Autodesk Inventor part; units mm, degrees
(part 4 of 5)
  arc A1726 (38.138, -15.9154) -> (38.5736, -15.5159) centre (32.062, -8.8527) ccw
  arc A1727 (38.5736, -15.5159) -> (39.0378, -15.0415) centre (28.2371, -4.9387) ccw
  arc A1728 (39.4893, -14.5664) -> (39.0378, -15.0415) centre (69.1048, -43.1656) ccw
  arc A1729 (39.8856, -14.1661) -> (39.4893, -14.5664) centre (55.6999, -30.2207) ccw
  arc A1730 (40.2317, -13.8281) -> (39.8856, -14.1661) centre (79.9781, -54.8675) ccw
  arc A1731 (40.296, -13.8021) -> (40.2317, -13.8281) centre (40.296, -13.8945) ccw
  arc A1732 (40.3238, -13.8373) -> (40.296, -13.8021) centre (40.296, -13.8306) ccw
  arc A1733 (40.2361, -14.1843) -> (40.3238, -13.8373) centre (23.2158, -9.7) ccw
  arc A1734 (40.1155, -14.6043) -> (40.2361, -14.1843) centre (30.6472, -11.658) ccw
  arc A1735 (39.9532, -15.1035) -> (40.1155, -14.6043) centre (20.5263, -8.5085) ccw
  line L90 (39.9532, -15.1035) -> (39.5114, -16.4048)
  line L91 (39.5114, -16.4048) -> (37.0556, -16.4773)
  arc A1736 (34.2634, -16.5112) -> (37.0556, -16.4773) centre (34.6839, 63.8924) ccw
  arc A1737 (33.9109, -16.1475) -> (34.2634, -16.5112) centre (34.2653, -16.1567) ccw
  arc A1738 (34.1876, -15.4924) -> (33.9109, -16.1475) centre (34.8846, -16.1728) ccw
  arc A1739 (37.1593, -12.4821) -> (34.1876, -15.4924) centre (301.3137, -276.224) ccw
  arc A1740 (37.1593, -12.4821) -> (38.6012, -11.0205) centre (-83.7235, 108.212) ccw
  arc A1741 (38.6012, -11.0205) -> (39.8159, -9.7502) centre (-27.3085, 53.2232) ccw
  arc A1742 (39.8159, -9.7502) -> (40.8574, -8.6344) centre (-176.4109, 193.1049) ccw
  arc A1743 (40.8574, -8.6344) -> (40.9209, -8.4725) centre (40.683, -8.4725) ccw
  arc A1744 (40.9209, -8.4725) -> (40.8525, -8.4427) centre (40.8802, -8.4725) ccw
  arc A1745 (40.8525, -8.4427) -> (39.7666, -9.4542) centre (214.237, -195.6686) ccw
  arc A1746 (39.7666, -9.4542) -> (38.4985, -10.6666) centre (99.0318, -72.7087) ccw
  arc A1747 (38.4985, -10.6666) -> (36.9912, -12.1544) centre (166.2662, -141.6192) ccw
  line L92 (36.9912, -12.1544) -> (33.0615, -16.0783)
  line L93 (33.0615, -16.0783) -> (31.7577, -15.4176)
  line L94 (31.7577, -15.4176) -> (30.454, -14.757)
  line L95 (30.454, -14.757) -> (32.403, -12.6971)
  arc A1748 (33.3514, -11.7342) -> (32.403, -12.6971) centre (56.8365, -35.8159) ccw
  arc A1749 (34.1156, -11.0538) -> (33.3514, -11.7342) centre (41.2243, -19.8071) ccw
  arc A1750 (34.7535, -10.5962) -> (34.1156, -11.0538) centre (38.2519, -16.147) ccw
  arc A1751 (35.297, -10.3468) -> (34.7535, -10.5962) centre (35.964, -12.5169) ccw
  arc A1752 (35.297, -10.3468) -> (35.6895, -10.225) centre (12.0441, 65.3116) ccw
  arc A1753 (35.6895, -10.225) -> (36.0874, -10.0994) centre (10.5624, 70.0447) ccw
  arc A1754 (36.0874, -10.0994) -> (36.4381, -9.9868) centre (13.3316, 61.3495) ccw
  arc A1755 (36.4381, -9.9868) -> (36.6604, -9.9126) centre (32.3763, 2.5531) ccw
  arc A1756 (36.7054, -9.9776) -> (36.6604, -9.9126) centre (36.6738, -9.9514) ccw
  arc A1757 (36.1561, -10.6219) -> (36.7054, -9.9776) centre (16.3124, 6.8533) ccw
  arc A1758 (35.3718, -11.4796) -> (36.1561, -10.6219) centre (12.8473, 9.9048) ccw
  arc A1759 (34.3562, -12.5291) -> (35.3718, -11.4796) centre (-20.1635, 41.2446) ccw
  arc A1760 (34.3562, -12.5291) -> (33.3301, -13.588) centre (93.5068, -70.8702) ccw
  arc A1761 (33.3301, -13.588) -> (32.509, -14.4785) centre (60.9355, -39.8655) ccw
  arc A1762 (32.509, -14.4785) -> (31.8583, -15.2176) centre (84.1452, -60.5934) ccw
  arc A1763 (31.8583, -15.2176) -> (31.8911, -15.2894) centre (31.8911, -15.246) ccw
  arc A1764 (31.8911, -15.2894) -> (32.059, -15.2242) centre (31.8911, -15.0404) ccw
  arc A1765 (32.059, -15.2242) -> (32.9062, -14.4424) centre (-48.4152, 72.8292) ccw
  arc A1766 (32.9062, -14.4424) -> (33.8794, -13.5112) centre (-1.8359, 22.8417) ccw
  arc A1767 (33.8794, -13.5112) -> (34.9854, -12.406) centre (-30.7449, 52.2666) ccw
  arc A1768 (36.9022, -10.5345) -> (34.9854, -12.406) centre (82.5718, -59.2267) ccw
  arc A1769 (38.4555, -9.2015) -> (36.9022, -10.5345) centre (52.7577, -27.4394) ccw
  arc A1770 (39.6868, -8.3356) -> (38.4555, -9.2015) centre (47.371, -20.5704) ccw
  arc A1771 (40.4694, -8.1054) -> (39.6868, -8.3356) centre (40.4864, -9.6088) ccw
  arc A1772 (40.657, -8.1316) -> (40.4694, -8.1054) centre (40.4766, -8.7387) ccw
  arc A1773 (40.8777, -8.2165) -> (40.657, -8.1316) centre (40.227, -9.5787) ccw
  arc A1774 (41.0953, -8.3415) -> (40.8777, -8.2165) centre (40.1633, -9.7121) ccw
  arc A1775 (41.275, -8.4902) -> (41.0953, -8.3415) centre (40.3973, -9.3679) ccw
  arc A1776 (31.7084, -10.6223) -> (31.7492, -10.5098) centre (31.5736, -10.5098) ccw
  arc A1777 (31.3694, -11.0202) -> (31.7084, -10.6223) centre (11.4621, 6.2854) ccw
  arc A1778 (30.9517, -11.4825) -> (31.3694, -11.0202) centre (19.0472, -0.3084) ccw
  arc A1779 (30.4563, -11.9971) -> (30.9517, -11.4825) centre (10.4353, 7.7752) ccw
  arc A1780 (30.4563, -11.9971) -> (29.9776, -12.4996) centre (44.1557, -25.5264) ccw
  arc A1781 (29.9776, -12.4996) -> (29.6159, -12.9217) centre (35.8733, -17.9166) ccw
  arc A1782 (29.6159, -12.9217) -> (29.3775, -13.2419) centre (34.2682, -16.6353) ccw
  arc A1783 (29.3775, -13.2419) -> (29.4112, -13.3063) centre (29.4112, -13.2653) ccw
  arc A1784 (29.4112, -13.3063) -> (29.5618, -13.2534) centre (29.4112, -13.0654) ccw
  arc A1785 (29.5618, -13.2534) -> (29.9818, -12.9058) centre (18.97, -0.0287) ccw
  arc A1786 (29.9818, -12.9058) -> (30.4717, -12.4653) centre (21.3967, -2.8664) ccw
  arc A1787 (30.4717, -12.4653) -> (31.0055, -11.9429) centre (15.5086, 3.3615) ccw
  arc A1788 (31.7567, -11.2175) -> (31.0055, -11.9429) centre (46.6591, -27.402) ccw
  arc A1789 (32.2629, -10.8345) -> (31.7567, -11.2175) centre (33.9908, -13.6438) ccw
  arc A1790 (32.7105, -10.6444) -> (32.2629, -10.8345) centre (33.1169, -12.223) ccw
  arc A1791 (33.2222, -10.5796) -> (32.7105, -10.6444) centre (33.2222, -12.6321) ccw
  line L96 (33.2222, -10.5796) -> (34.0925, -10.5796)
  line L97 (34.0925, -10.5796) -> (32.1196, -12.5641)
  arc A1792 (31.3452, -13.3188) -> (32.1196, -12.5641) centre (7.8652, 11.548) ccw
  arc A1793 (30.6521, -13.9417) -> (31.3452, -13.3188) centre (18.3556, 0.438) ccw
  arc A1794 (30.058, -14.4365) -> (30.6521, -13.9417) centre (11.4069, 8.5638) ccw
  arc A1795 (29.8944, -14.4669) -> (30.058, -14.4365) centre (29.9482, -14.301) ccw
  arc A1796 (29.7762, -14.393) -> (29.8944, -14.4669) centre (29.9829, -14.1937) ccw
  arc A1797 (29.6203, -14.2122) -> (29.7762, -14.393) centre (31.3225, -12.9019) ccw
  arc A1798 (29.459, -13.9774) -> (29.6203, -14.2122) centre (31.6971, -12.6135) ccw
  arc A1799 (29.3154, -13.7147) -> (29.459, -13.9774) centre (32.1853, -12.316) ccw
  arc A1800 (29.1585, -13.0704) -> (29.3154, -13.7147) centre (30.7144, -13.0329) ccw
  arc A1801 (29.236, -12.262) -> (29.1585, -13.0704) centre (32.5603, -12.9883) ccw
  arc A1802 (29.5153, -11.4435) -> (29.236, -12.262) centre (32.9572, -13.075) ccw
  arc A1803 (29.9598, -10.7655) -> (29.5153, -11.4435) centre (32.1847, -12.7089) ccw
  arc A1804 (30.3493, -10.5014) -> (29.9598, -10.7655) centre (30.657, -11.3745) ccw
  arc A1805 (30.9913, -10.344) -> (30.3493, -10.5014) centre (31.4668, -13.6724) ccw
  arc A1806 (31.5755, -10.3233) -> (30.9913, -10.344) centre (31.3801, -13.0655) ccw
  arc A1807 (31.7492, -10.5098) -> (31.5755, -10.3233) centre (31.5622, -10.5098) ccw
  arc A1808 (46.7213, -8.0425) -> (46.3577, -8.3987) centre (47.4846, -9.1857) ccw
  arc A1809 (46.3577, -8.3987) -> (46.1142, -8.8903) centre (47.8654, -9.4516) ccw
  arc A1810 (46.1142, -8.8903) -> (46.0266, -9.4315) centre (47.8632, -9.4509) ccw
  arc A1811 (46.0266, -9.4315) -> (46.1158, -9.9317) centre (47.3936, -9.4459) ccw
  arc A1812 (46.1158, -9.9317) -> (46.4364, -10.4266) centre (47.4287, -9.4326) ccw
  arc A1813 (46.4364, -10.4266) -> (46.9984, -10.8648) centre (48.4994, -8.36) ccw
  arc A1814 (46.9984, -10.8648) -> (47.6192, -11.1375) centre (48.3863, -8.5487) ccw
  arc A1815 (47.6192, -11.1375) -> (48.1096, -11.1265) centre (47.8471, -10.3684) ccw
  arc A1816 (48.1096, -11.1265) -> (48.8176, -10.6423) centre (47.5768, -9.5875) ccw
  arc A1817 (48.8176, -10.6423) -> (49.2477, -9.8286) centre (47.1986, -9.266) ccw
  arc A1818 (49.2477, -9.8286) -> (49.2809, -8.9454) centre (47.3812, -9.3162) ccw
  arc A1819 (49.2809, -8.9454) -> (48.8957, -8.2631) centre (48.0631, -9.1831) ccw
  arc A1820 (48.8957, -8.2631) -> (48.4527, -8.0069) centre (48.077, -9.1676) ccw
  arc A1821 (48.4527, -8.0069) -> (47.8163, -7.8732) centre (47.5061, -10.9318) ccw
  arc A1822 (47.8163, -7.8732) -> (47.1752, -7.8767) centre (47.5119, -10.8742) ccw
  arc A1823 (47.1752, -7.8767) -> (46.7213, -8.0425) centre (47.2894, -8.8933) ccw
  arc A1824 (48.7931, -8.8222) -> (48.5558, -8.3982) centre (47.9232, -9.0307) ccw
  arc A1825 (48.8362, -9.4068) -> (48.7931, -8.8222) centre (47.0228, -9.2466) ccw
  arc A1826 (48.6892, -9.9974) -> (48.8362, -9.4068) centre (46.8825, -9.2342) ccw
  arc A1827 (48.3754, -10.4393) -> (48.6892, -9.9974) centre (47.5338, -9.5093) ccw
  arc A1828 (48.087, -10.6623) -> (48.3754, -10.4393) centre (46.7951, -8.6931) ccw
  arc A1829 (47.8597, -10.7406) -> (48.087, -10.6623) centre (47.8192, -10.254) ccw
  arc A1830 (47.6028, -10.7066) -> (47.8597, -10.7406) centre (47.8092, -10.1344) ccw
  arc A1831 (47.198, -10.5374) -> (47.6028, -10.7066) centre (49.0977, -6.5617) ccw
  arc A1832 (46.9119, -10.3629) -> (47.198, -10.5374) centre (47.9066, -9.0545) ccw
  arc A1833 (46.6708, -10.1357) -> (46.9119, -10.3629) centre (47.8627, -9.1122) ccw
  arc A1834 (46.4984, -9.8815) -> (46.6708, -10.1357) centre (47.6992, -9.2526) ccw
  arc A1835 (46.4164, -9.6272) -> (46.4984, -9.8815) centre (47.1954, -9.5165) ccw
  arc A1836 (46.5581, -8.8824) -> (46.4164, -9.6272) centre (47.5771, -9.4622) ccw
  arc A1837 (47.1366, -8.3016) -> (46.5581, -8.8824) centre (47.9132, -9.6534) ccw
  arc A1838 (47.9043, -8.113) -> (47.1366, -8.3016) centre (47.8475, -9.5391) ccw
  arc A1839 (48.5558, -8.3982) -> (47.9043, -8.113) centre (47.8655, -9.0885) ccw
  arc A1840 (-50.4415, -11.5045) -> (-50.7344, -11.3634) centre (-51.3001, -12.9124) ccw
  arc A1841 (-50.2214, -11.6868) -> (-50.4415, -11.5045) centre (-50.9596, -12.354) ccw
  arc A1842 (-50.0815, -11.9045) -> (-50.2214, -11.6868) centre (-50.8108, -12.2195) ccw
  arc A1843 (-50.024, -12.1495) -> (-50.0815, -11.9045) centre (-50.737, -12.1877) ccw
  arc A1844 (-50.024, -12.1495) -> (-50.0042, -12.4881) centre (-14.2029, -10.2317) ccw
  arc A1845 (-50.0042, -12.4881) -> (-49.98, -12.5211) centre (-49.9665, -12.4857) ccw
  arc A1846 (-49.98, -12.5211) -> (-49.9513, -12.5064) centre (-49.9722, -12.5008) ccw
  arc A1847 (-49.9513, -12.5064) -> (-49.8731, -12.2072) centre (-74.3795, -5.9632) ccw
  arc A1848 (-49.8731, -12.2072) -> (-49.9017, -11.8206) centre (-50.4639, -12.0567) ccw
  arc A1849 (-49.9017, -11.8206) -> (-50.1607, -11.4431) centre (-50.9451, -12.2587) ccw
  arc A1850 (-50.1607, -11.4431) -> (-50.5726, -11.1738) centre (-51.0791, -12.3981) ccw
  arc A1851 (-50.5726, -11.1738) -> (-51.0297, -11.0949) centre (-50.9763, -12.1494) ccw
  arc A1852 (-51.0297, -11.0949) -> (-51.1035, -11.1276) centre (-51.024, -11.2076) ccw
  arc A1853 (-51.1035, -11.1276) -> (-51.1023, -11.1819) centre (-51.0771, -11.1541) ccw
  arc A1854 (-51.1023, -11.1819) -> (-50.9743, -11.2658) centre (-50.7742, -10.8211) ccw
  arc A1855 (-50.9743, -11.2658) -> (-50.7344, -11.3634) centre (-49.511, -8.0137) ccw
  arc A1856 (-8.6486, -11.8882) -> (-9.2341, -12.3218) centre (-7.6704, -13.8214) ccw
  arc A1857 (-9.2341, -12.3218) -> (-9.814, -13.0398) centre (-5.3124, -16.0826) ccw
  arc A1858 (-9.814, -13.0398) -> (-10.2534, -13.8266) centre (-5.4203, -16.0096) ccw
  arc A1859 (-10.2534, -13.8266) -> (-10.3912, -14.4664) centre (-8.8369, -14.4664) ccw
  arc A1860 (-10.3912, -14.4664) -> (-10.2891, -15.198) centre (-7.718, -14.4664) ccw
  arc A1861 (-10.2891, -15.198) -> (-9.9826, -15.9905) centre (-5.8322, -13.9298) ccw
  arc A1862 (-9.9826, -15.9905) -> (-9.5475, -16.6938) centre (-6.0016, -14.0139) ccw
  arc A1863 (-9.5475, -16.6938) -> (-9.058, -17.1515) centre (-7.9836, -15.5118) ccw
  arc A1864 (-9.058, -17.1515) -> (-8.277, -17.522) centre (-7.3254, -14.5073) ccw
  arc A1865 (-8.277, -17.522) -> (-7.3739, -17.6972) centre (-7.0611, -13.67) ccw
  arc A1866 (-7.3739, -17.6972) -> (-6.476, -17.6621) centre (-7.0747, -13.8454) ccw
  arc A1867 (-6.476, -17.6621) -> (-5.7108, -17.4116) centre (-6.8656, -15.1784) ccw
  arc A1868 (-5.7108, -17.4116) -> (-4.7772, -16.6666) centre (-7.1175, -14.6913) ccw
  arc A1869 (-4.7772, -16.6666) -> (-4.1582, -15.5951) centre (-7.4602, -14.4021) ccw
  arc A1870 (-4.1582, -15.5951) -> (-3.9541, -14.3873) centre (-7.3882, -14.4281) ccw
  arc A1871 (-3.9541, -14.3873) -> (-4.2077, -13.2514) centre (-6.7741, -14.4208) ccw
  arc A1872 (-4.2077, -13.2514) -> (-4.9315, -12.3561) centre (-6.3063, -14.2076) ccw
  arc A1873 (-4.9315, -12.3561) -> (-6.1103, -11.7598) centre (-7.2532, -15.4829) ccw
  arc A1874 (-6.1103, -11.7598) -> (-7.4534, -11.5815) centre (-7.3143, -15.6818) ccw
  arc A1875 (-7.4534, -11.5815) -> (-8.6486, -11.8882) centre (-7.3564, -14.4419) ccw
  arc A1876 (-4.7478, -13.2418) -> (-5.2538, -12.6927) centre (-11.7267, -19.1656) ccw
  arc A1877 (-4.5289, -13.6208) -> (-4.7478, -13.2418) centre (-5.6794, -14.0326) ccw
  arc A1878 (-4.4572, -14.0533) -> (-4.5289, -13.6208) centre (-5.6855, -14.0347) ccw
  arc A1879 (-4.4988, -14.8023) -> (-4.4572, -14.0533) centre (-13.7563, -13.9127) ccw
  arc A1880 (-4.6776, -15.7395) -> (-4.4988, -14.8023) centre (-9.6283, -14.3094) ccw
  arc A1881 (-5.0155, -16.4236) -> (-4.6776, -15.7395) centre (-6.7527, -15.1401) ccw
  arc A1882 (-5.5524, -16.9186) -> (-5.0155, -16.4236) centre (-6.5733, -15.2726) ccw
  arc A1883 (-6.3311, -17.2823) -> (-5.5524, -16.9186) centre (-7.4731, -13.8219) ccw
  arc A1884 (-7.6809, -17.3654) -> (-6.3311, -17.2823) centre (-7.1637, -14.7594) ccw
  arc A1885 (-8.8938, -16.7727) -> (-7.6809, -17.3654) centre (-7.1671, -14.7764) ccw
  arc A1886 (-9.6718, -15.6457) -> (-8.8938, -16.7727) centre (-7.1073, -14.7072) ccw
  arc A1887 (-9.8229, -14.2621) -> (-9.6718, -15.6457) centre (-6.9455, -14.648) ccw
  arc A1888 (-9.5204, -13.2273) -> (-9.8229, -14.2621) centre (-6.2735, -14.7382) ccw
  arc A1889 (-8.9428, -12.4702) -> (-9.5204, -13.2273) centre (-7.5078, -14.1638) ccw
  arc A1890 (-8.0839, -12.0074) -> (-8.9428, -12.4702) centre (-7.4209, -14.2664) ccw
  arc A1891 (-6.958, -11.8347) -> (-8.0839, -12.0074) centre (-6.8769, -16.1196) ccw
  arc A1892 (-6.5115, -11.8746) -> (-6.958, -11.8347) centre (-6.9186, -13.9142) ccw
  arc A1893 (-6.1183, -12.01) -> (-6.5115, -11.8746) centre (-6.8146, -13.393) ccw
  arc A1894 (-5.7208, -12.269) -> (-6.1183, -12.01) centre (-7.0812, -13.9226) ccw
  arc A1895 (-5.2538, -12.6927) -> (-5.7208, -12.269) centre (-9.8548, -17.2937) ccw
  arc A1896 (21.7067, -11.8336) -> (21.1335, -12.2767) centre (22.6164, -13.6027) ccw
  arc A1897 (21.1335, -12.2767) -> (20.6054, -13) centre (24.5132, -15.2988) ccw
  arc A1898 (20.6054, -13) -> (20.2257, -13.8207) centre (24.5692, -15.3317) ccw
  arc A1899 (20.2257, -13.8207) -> (20.1023, -14.561) centre (22.3265, -14.5515) ccw
  arc A1900 (20.1023, -14.561) -> (20.547, -16.1601) centre (23.248, -14.5476) ccw
  arc A1901 (20.547, -16.1601) -> (21.7473, -17.332) centre (23.357, -14.4825) ccw
  arc A1902 (21.7473, -17.332) -> (23.3658, -17.7519) centre (23.3447, -14.5043) ccw
  arc A1903 (23.3658, -17.7519) -> (24.9522, -17.3008) centre (23.3457, -14.6664) ccw
  arc A1904 (24.9522, -17.3008) -> (25.9352, -16.3533) centre (23.3193, -14.623) ccw
  arc A1905 (25.9352, -16.3533) -> (26.4072, -15.0895) centre (23.4348, -14.6994) ccw
  arc A1906 (26.4072, -15.0895) -> (26.2808, -13.7295) centre (23.3481, -14.688) ccw
  arc A1907 (26.2808, -13.7295) -> (25.5804, -12.5135) centre (23.0306, -14.7918) ccw
  arc A1908 (25.5804, -12.5135) -> (25.1593, -12.105) centre (22.5116, -15.2555) ccw
  arc A1909 (25.1593, -12.105) -> (24.7721, -11.8685) centre (24.1861, -13.263) ccw
  arc A1910 (24.7721, -11.8685) -> (24.2922, -11.7358) centre (24.0164, -13.667) ccw
  arc A1911 (24.2922, -11.7358) -> (23.5487, -11.6599) centre (22.9749, -20.9586) ccw
  arc A1912 (23.5487, -11.6599) -> (22.9979, -11.647) centre (23.1056, -18.8402) ccw
  arc A1913 (22.9979, -11.647) -> (22.4536, -11.6767) centre (23.1011, -18.543) ccw
  arc A1914 (22.4536, -11.6767) -> (21.9858, -11.7397) centre (23.0095, -17.571) ccw
  arc A1915 (21.9858, -11.7397) -> (21.7067, -11.8336) centre (22.1555, -12.7063) ccw
  arc A1916 (24.9716, -12.4173) -> (24.4203, -12.0607) centre (23.8629, -13.527) ccw
  arc A1917 (25.5115, -13.0765) -> (24.9716, -12.4173) centre (21.9442, -15.4472) ccw
  arc A1918 (25.9145, -13.8372) -> (25.5115, -13.0765) centre (21.8957, -15.4795) ccw
  arc A1919 (26.0469, -14.5082) -> (25.9145, -13.8372) centre (24.2654, -14.5111) ccw
  arc A1920 (25.9247, -15.2823) -> (26.0469, -14.5082) centre (23.5599, -14.5122) ccw
  arc A1921 (25.5627, -16.0554) -> (25.9247, -15.2823) centre (22.62, -14.2061) ccw
  arc A1922 (25.0239, -16.7157) -> (25.5627, -16.0554) centre (22.6297, -14.2122) ccw
  arc A1923 (24.3818, -17.1579) -> (25.0239, -16.7157) centre (23.3328, -14.9474) ccw
  arc A1924 (23.0524, -17.4187) -> (24.3818, -17.1579) centre (23.2049, -14.6779) ccw
  arc A1925 (21.801, -16.9988) -> (23.0524, -17.4187) centre (23.1908, -14.9316) ccw
  arc A1926 (20.9144, -15.9847) -> (21.801, -16.9988) centre (23.2601, -14.8286) ccw
  arc A1927 (20.5944, -14.6114) -> (20.9144, -15.9847) centre (23.7007, -14.6114) ccw
  arc A1928 (20.6315, -13.9946) -> (20.5944, -14.6114) centre (25.7415, -14.6114) ccw
  arc A1929 (20.7507, -13.5536) -> (20.6315, -13.9946) centre (22.2124, -14.1855) ccw
  arc A1930 (20.9941, -13.1527) -> (20.7507, -13.5536) centre (22.3204, -14.2321) ccw
  arc A1931 (21.4372, -12.6618) -> (20.9941, -13.1527) centre (26.0121, -17.2367) ccw
  arc A1932 (22.1134, -12.1257) -> (21.4372, -12.6618) centre (24.0937, -15.3183) ccw
  arc A1933 (22.8041, -11.8522) -> (22.1134, -12.1257) centre (23.2181, -13.9066) ccw
  arc A1934 (23.5572, -11.834) -> (22.8041, -11.8522) centre (23.2324, -13.9776) ccw
  arc A1935 (24.4203, -12.0607) -> (23.5572, -11.834) centre (22.9282, -15.9853) ccw
  arc A1936 (-61.0775, -12.1557) -> (-61.2696, -12.3511) centre (-60.5776, -12.8394) ccw
  arc A1937 (-61.2696, -12.3511) -> (-61.4156, -12.6202) centre (-60.2017, -13.1046) ccw
  arc A1938 (-61.4156, -12.6202) -> (-61.5073, -12.9461) centre (-59.9224, -13.2161) ccw
  arc A1939 (-61.5073, -12.9461) -> (-61.538, -13.3098) centre (-59.3719, -13.3098) ccw
  arc A1940 (-61.538, -13.3098) -> (-61.2621, -14.2496) centre (-59.7999, -13.3098) ccw
  arc A1941 (-61.2621, -14.2496) -> (-60.5238, -14.8803) centre (-59.8459, -13.3394) ccw
  arc A1942 (-60.5238, -14.8803) -> (-59.5734, -14.9904) centre (-59.8701, -13.3944) ccw
  arc A1943 (-59.5734, -14.9904) -> (-58.7287, -14.5457) centre (-59.8678, -13.4066) ccw
  arc A1944 (-58.7287, -14.5457) -> (-58.283, -13.4563) centre (-59.8049, -13.4695) ccw
  arc A1945 (-58.283, -13.4563) -> (-58.7393, -12.3545) centre (-59.8745, -13.4701) ccw
  arc A1946 (-58.7393, -12.3545) -> (-59.875, -11.8196) centre (-60.0311, -13.624) ccw
  arc A1947 (-59.875, -11.8196) -> (-61.0775, -12.1557) centre (-60.0282, -13.5907) ccw
  arc A1948 (-58.6887, -13.1367) -> (-58.8881, -12.5872) centre (-59.8097, -13.2327) ccw
  arc A1949 (-58.755, -13.7936) -> (-58.6887, -13.1367) centre (-60.4668, -13.2889) ccw
  arc A1950 (-59.0517, -14.3667) -> (-58.755, -13.7936) centre (-60.3851, -13.313) ccw
  arc A1951 (-59.5052, -14.6801) -> (-59.0517, -14.3667) centre (-59.7898, -13.7835) ccw
  arc A1952 (-60.0271, -14.6894) -> (-59.5052, -14.6801) centre (-59.7818, -13.8087) ccw
  arc A1953 (-60.6031, -14.4198) -> (-60.0271, -14.6894) centre (-59.5107, -12.8359) ccw
  arc A1954 (-61.0522, -13.9824) -> (-60.6031, -14.4198) centre (-59.5411, -12.8801) ccw
  arc A1955 (-61.2075, -13.506) -> (-61.0522, -13.9824) centre (-60.3992, -13.506) ccw
  arc A1956 (-60.9619, -12.7146) -> (-61.2075, -13.506) centre (-59.8099, -13.506) ccw
  arc A1957 (-60.3098, -12.1948) -> (-60.9619, -12.7146) centre (-59.7831, -13.5244) ccw
  arc A1958 (-59.5167, -12.1481) -> (-60.3098, -12.1948) centre (-59.8425, -13.3744) ccw
  arc A1959 (-58.8881, -12.5872) -> (-59.5167, -12.1481) centre (-59.8037, -13.2285) ccw
  arc A1960 (-52.0358, -12.548) -> (-52.0178, -12.6484) centre (-51.7463, -12.548) ccw
  arc A1961 (-52.0178, -12.6484) -> (-51.9638, -12.7572) centre (-51.4817, -12.4501) ccw
  arc A1962 (-51.9638, -12.7572) -> (-51.8845, -12.8575) centre (-51.4358, -12.4209) ccw
  arc A1963 (-51.8845, -12.8575) -> (-51.7908, -12.9327) centre (-51.5327, -12.5152) ccw
  arc A1964 (-51.7908, -12.9327) -> (-51.7071, -12.961) centre (-51.688, -12.7665) ccw
  arc A1965 (-51.7071, -12.961) -> (-51.6576, -12.9314) centre (-51.7024, -12.9127) ccw
  arc A1966 (-51.6576, -12.9314) -> (-51.6499, -12.8432) centre (-51.7923, -12.8751) ccw
  arc A1967 (-51.6499, -12.8432) -> (-51.6933, -12.6995) centre (-52.6572, -13.0693) ccw
  arc A1968 (-51.6933, -12.6995) -> (-51.814, -12.4337) centre (-53.9686, -13.5725) ccw
  arc A1969 (-51.814, -12.4337) -> (-51.9264, -12.329) centre (-52.0211, -12.5432) ccw
  arc A1970 (-51.9264, -12.329) -> (-52.0066, -12.3648) centre (-51.9503, -12.3832) ccw
  arc A1971 (-52.0066, -12.3648) -> (-52.0358, -12.548) centre (-51.4456, -12.548) ccw
  arc A1972 (-51.0907, -13.2277) -> (-50.9552, -13.2664) centre (-50.8353, -12.5895) ccw
  arc A1973 (-50.9552, -13.2664) -> (-50.817, -13.2757) centre (-50.8434, -12.6348) ccw
  arc A1974 (-50.817, -13.2757) -> (-50.6967, -13.2561) centre (-50.8378, -12.7693) ccw
  arc A1975 (-50.6967, -13.2561) -> (-50.6156, -13.2082) centre (-50.7493, -13.0745) ccw
  arc A1976 (-50.6156, -13.2082) -> (-50.6042, -13.1539) centre (-50.6515, -13.1722) ccw
  arc A1977 (-50.6042, -13.1539) -> (-50.6494, -13.1081) centre (-50.6794, -13.183) ccw
  arc A1978 (-50.6494, -13.1081) -> (-50.7684, -13.0807) centre (-50.7973, -13.4778) ccw
  arc A1979 (-50.7684, -13.0807) -> (-50.941, -13.078) centre (-50.8786, -14.5925) ccw
  arc A1980 (-50.941, -13.078) -> (-51.126, -13.0926) centre (-50.8399, -15.5323) ccw
  arc A1981 (-51.126, -13.0926) -> (-51.1983, -13.1276) centre (-51.1117, -13.2142) ccw
  arc A1982 (-51.1983, -13.1276) -> (-51.194, -13.1728) centre (-51.1775, -13.1485) ccw
  arc A1983 (-51.194, -13.1728) -> (-51.0907, -13.2277) centre (-50.8892, -12.7241) ccw
  arc A1984 (54.3957, -29.633) -> (53.8937, -29.9822) centre (57.8749, -35.1695) ccw
  arc A1985 (53.8937, -29.9822) -> (53.5183, -30.3224) centre (55.7859, -32.4477) ccw
  arc A1986 (53.5183, -30.3224) -> (53.3673, -30.5575) centre (54.0814, -30.8502) ccw
  arc A1987 (53.3673, -30.5575) -> (53.4348, -30.6582) centre (53.4348, -30.5852) ccw
  arc A1988 (53.4348, -30.6582) -> (53.52, -30.6333) centre (53.4348, -30.5004) ccw
  arc A1989 (53.52, -30.6333) -> (53.6954, -30.5135) centre (51.5661, -27.5843) ccw
  arc A1990 (53.6954, -30.5135) -> (53.8992, -30.3542) centre (51.504, -27.4989) ccw
  arc A1991 (53.8992, -30.3542) -> (54.1126, -30.1655) centre (50.3806, -26.1597) ccw
  arc A1992 (55.6105, -29.4753) -> (54.1126, -30.1655) centre (55.909, -32.0938) ccw
  arc A1993 (57.241, -29.8019) -> (55.6105, -29.4753) centre (55.9181, -32.1732) ccw
  arc A1994 (58.4128, -31.0329) -> (57.241, -29.8019) centre (55.8452, -32.3038) ccw
  arc A1995 (58.6904, -32.7194) -> (58.4128, -31.0329) centre (55.7911, -32.3306) ccw
  arc A1996 (58.4067, -33.7014) -> (58.6904, -32.7194) centre (55.2548, -32.2586) ccw
  arc A1997 (57.8674, -34.4181) -> (58.4067, -33.7014) centre (56.5025, -32.8298) ccw
  arc A1998 (57.0722, -34.849) -> (57.8674, -34.4181) centre (56.4745, -32.7972) ccw
  arc A1999 (56.041, -34.9962) -> (57.0722, -34.849) centre (56.041, -31.3092) ccw
  arc A2000 (55.3527, -34.964) -> (56.041, -34.9962) centre (56.041, -27.61) ccw
  arc A2001 (54.8936, -34.8559) -> (55.3527, -34.964) centre (55.5124, -33.2584) ccw
  arc A2002 (54.4997, -34.6315) -> (54.8936, -34.8559) centre (55.448, -33.4246) ccw
  arc A2003 (54.035, -34.2192) -> (54.4997, -34.6315) centre (57.7167, -30.5374) ccw
  arc A2004 (53.617, -33.7476) -> (54.035, -34.2192) centre (57.744, -30.5101) ccw
  arc A2005 (53.3941, -33.3508) -> (53.617, -33.7476) centre (54.7882, -32.8288) ccw
  arc A2006 (53.2884, -32.8797) -> (53.3941, -33.3508) centre (55.0414, -32.734) ccw
  arc A2007 (53.2579, -32.1438) -> (53.2884, -32.8797) centre (62.1467, -32.1438) ccw
  arc A2008 (53.2579, -32.1438) -> (53.2459, -31.6008) centre (40.9961, -32.1438) ccw
  arc A2009 (53.2459, -31.6008) -> (53.2019, -31.2714) centre (51.3667, -31.6841) ccw
  arc A2010 (53.2019, -31.2714) -> (53.1293, -31.1668) centre (53.0367, -31.3086) ccw
  arc A2011 (53.1293, -31.1668) -> (53.0425, -31.1856) centre (53.0952, -31.219) ccw
  arc A2012 (53.0425, -31.1856) -> (52.8122, -32.0857) centre (54.3121, -31.9899) ccw
  arc A2013 (52.8122, -32.0857) -> (53.0721, -33.2523) centre (56.6656, -31.8396) ccw
  arc A2014 (53.0721, -33.2523) -> (53.7034, -34.3497) centre (57.0808, -31.6763) ccw
  arc A2015 (53.7034, -34.3497) -> (54.562, -35.0509) centre (55.7275, -32.7475) ccw
  arc A2016 (54.562, -35.0509) -> (55.7936, -35.3677) centre (55.8976, -32.4114) ccw
  arc A2017 (55.7936, -35.3677) -> (57.0675, -35.1472) centre (55.9044, -32.2185) ccw
  arc A2018 (57.0675, -35.1472) -> (58.1619, -34.4282) centre (55.8703, -32.1325) ccw
  arc A2019 (58.1619, -34.4282) -> (58.8838, -33.3345) centre (55.864, -32.1263) ccw
  arc A2020 (58.8838, -33.3345) -> (59.1079, -32.7077) centre (50.5845, -30.0138) ccw
  arc A2021 (59.1079, -32.7077) -> (59.1718, -32.3059) centre (57.797, -32.2934) ccw
  arc A2022 (59.1718, -32.3059) -> (59.1146, -31.907) centre (57.836, -32.2937) ccw
  arc A2023 (59.1146, -31.907) -> (58.9024, -31.2943) centre (51.2905, -34.2732) ccw
  arc A2024 (58.9024, -31.2943) -> (58.7043, -30.8741) centre (55.7009, -32.5472) ccw
  arc A2025 (58.7043, -30.8741) -> (58.4351, -30.4451) centre (54.4672, -33.2344) ccw
  arc A2026 (58.4351, -30.4451) -> (58.1399, -30.0696) centre (54.7798, -33.0147) ccw
  arc A2027 (58.1399, -30.0696) -> (57.8652, -29.8188) centre (56.8787, -31.175) ccw
  arc A2028 (57.8652, -29.8188) -> (57.0705, -29.4158) centre (56.2154, -32.0869) ccw
  arc A2029 (57.0705, -29.4158) -> (56.1262, -29.2423) centre (55.9253, -32.993) ccw
  arc A2030 (56.1262, -29.2423) -> (55.184, -29.3146) centre (55.9314, -32.8794) ccw
  arc A2031 (55.184, -29.3146) -> (54.3957, -29.633) centre (55.6789, -31.6749) ccw
  arc A2032 (54.8437, -31.1688) -> (54.6468, -31.385) centre (56.0572, -32.4713) ccw
  arc A2033 (54.6468, -31.385) -> (54.508, -31.6124) centre (55.623, -32.1368) ccw
  arc A2034 (54.508, -31.6124) -> (54.4429, -31.817) centre (55.25, -31.9614) ccw
  arc A2035 (54.4429, -31.817) -> (54.4705, -31.9622) centre (54.6464, -31.8534) ccw
  arc A2036 (54.4705, -31.9622) -> (54.5564, -32.072) centre (55.0097, -31.6289) ccw
  arc A2037 (54.5564, -32.072) -> (54.6292, -32.0918) centre (54.6096, -32.0199) ccw
  arc A2038 (54.6292, -32.0918) -> (54.694, -32.0375) centre (54.6026, -31.994) ccw
  arc A2039 (54.694, -32.0375) -> (54.7524, -31.8854) centre (53.7388, -31.5836) ccw
  arc A2040 (54.8213, -31.7254) -> (54.7524, -31.8854) centre (55.468, -32.0985) ccw
  arc A2041 (54.9428, -31.5404) -> (54.8213, -31.7254) centre (56.4738, -32.6787) ccw
  arc A2042 (55.0927, -31.3609) -> (54.9428, -31.5404) centre (56.5996, -32.7723) ccw
  arc A2043 (55.2502, -31.2159) -> (55.0927, -31.3609) centre (56.152, -32.3531) ccw
  arc A2044 (56.1588, -30.9578) -> (55.2502, -31.2159) centre (56.0152, -32.1805) ccw
  arc A2045 (56.9827, -31.4194) -> (56.1588, -30.9578) centre (56.0152, -32.1802) ccw
  arc A2046 (57.2607, -32.3506) -> (56.9827, -31.4194) centre (55.9431, -32.2369) ccw
  arc A2047 (56.828, -33.2226) -> (57.2607, -32.3506) centre (55.9353, -32.2362) ccw
  arc A2048 (56.3195, -33.539) -> (56.828, -33.2226) centre (55.6993, -31.9754) ccw
  arc A2049 (55.7955, -33.6028) -> (56.3195, -33.539) centre (55.9357, -32.5715) ccw
  arc A2050 (55.2888, -33.4009) -> (55.7955, -33.6028) centre (55.9475, -32.4845) ccw
  arc A2051 (54.831, -32.9511) -> (55.2888, -33.4009) centre (56.5156, -31.6943) ccw
  arc A2052 (54.831, -32.9511) -> (54.6347, -32.71) centre (51.8763, -35.1556) ccw
  arc A2053 (54.6347, -32.71) -> (54.4695, -32.5607) centre (53.8807, -33.3785) ccw
  arc A2054 (54.4695, -32.5607) -> (54.3659, -32.5283) centre (54.369, -32.7003) ccw
  arc A2055 (54.3659, -32.5283) -> (54.3145, -32.5793) centre (54.3668, -32.5806) ccw
  arc A2056 (54.3145, -32.5793) -> (54.4492, -32.9991) centre (54.9832, -32.5963) ccw
  arc A2057 (54.4492, -32.9991) -> (54.8815, -33.4358) centre (56.2855, -31.6138) ccw
  arc A2058 (54.8815, -33.4358) -> (55.4506, -33.7683) centre (56.4608, -31.3863) ccw
  arc A2059 (55.4506, -33.7683) -> (56.0035, -33.8807) centre (56.0035, -32.4647) ccw
  arc A2060 (56.0035, -33.8807) -> (56.8949, -33.5923) centre (56.0035, -32.3588) ccw
  arc A2061 (56.8949, -33.5923) -> (57.4755, -32.8299) centre (55.9269, -32.2529) ccw
  arc A2062 (57.4755, -32.8299) -> (57.5301, -31.8836) centre (55.9678, -32.2682) ccw
  arc A2063 (57.5301, -31.8836) -> (57.0369, -31.107) centre (56.1287, -32.2286) ccw
  arc A2064 (57.0369, -31.107) -> (56.4843, -30.7816) centre (55.6733, -32.791) ccw
  arc A2065 (56.4843, -30.7816) -> (55.9205, -30.6803) centre (55.9599, -32.0809) ccw
  arc A2066 (55.9205, -30.6803) -> (55.3668, -30.8134) centre (55.9594, -32.0608) ccw
  arc A2067 (55.3668, -30.8134) -> (54.8437, -31.1688) centre (56.2555, -32.6841) ccw
  arc A2068 (-30.8266, -35.3804) -> (-31.1513, -35.5128) centre (-30.306, -37.1226) ccw
  arc A2069 (-31.1513, -35.5128) -> (-31.5276, -35.7353) centre (-29.141, -39.3412) ccw
  arc A2070 (-31.5276, -35.7353) -> (-31.8936, -36.0046) centre (-29.0077, -39.5428) ccw
  arc A2071 (-31.8936, -36.0046) -> (-32.1899, -36.2827) centre (-30.043, -38.2734) ccw
  arc A2072 (-32.1899, -36.2827) -> (-32.5168, -36.7013) centre (-29.8866, -38.4185) ccw
  arc A2073 (-32.5168, -36.7013) -> (-32.7048, -37.1046) centre (-31.2017, -37.5599) ccw
  arc A2074 (-32.7048, -37.1046) -> (-32.7977, -37.6091) centre (-30.5081, -37.77) ccw
  arc A2075 (-32.7977, -37.6091) -> (-32.8247, -38.3787) centre (-21.8439, -38.3787) ccw
  arc A2076 (-32.8247, -38.3787) -> (-32.7987, -39.1284) centre (-22.0069, -38.3787) ccw
  arc A2077 (-32.7987, -39.1284) -> (-32.7104, -39.6322) centre (-30.344, -38.9579) ccw
  arc A2078 (-32.7104, -39.6322) -> (-32.5372, -40.0258) centre (-31.1978, -39.2012) ccw
  arc A2079 (-32.5372, -40.0258) -> (-32.2475, -40.4045) centre (-30.5269, -38.7881) ccw
  arc A2080 (-32.2475, -40.4045) -> (-31.0733, -41.1687) centre (-30.0964, -38.3837) ccw
  arc A2081 (-31.0733, -41.1687) -> (-29.6241, -41.35) centre (-29.9293, -37.9074) ccw
  arc A2082 (-29.6241, -41.35) -> (-28.2415, -40.917) centre (-29.9239, -37.9692) ccw
  arc A2083 (-28.2415, -40.917) -> (-27.2521, -39.9616) centre (-29.6231, -38.4962) ccw
  arc A2084 (-27.2521, -39.9616) -> (-26.911, -39.3845) centre (-41.7402, -31.0074) ccw
  arc A2085 (-26.911, -39.3845) -> (-26.7824, -39.0706) centre (-28.0898, -38.7186) ccw
  arc A2086 (-26.7824, -39.0706) -> (-26.8107, -38.9105) centre (-26.9675, -39.0208) ccw
  arc A2087 (-26.8107, -38.9105) -> (-26.9497, -38.8384) centre (-26.9497, -39.0083) ccw
  arc A2088 (-26.9497, -38.8384) -> (-27.0437, -38.8848) centre (-26.9497, -38.9568) ccw
  arc A2089 (-27.0437, -38.8848) -> (-27.1776, -39.0818) centre (-25.3578, -40.1749) ccw
  arc A2090 (-27.1776, -39.0818) -> (-27.3182, -39.3496) centre (-24.9174, -40.4393) ccw
  arc A2091 (-27.3182, -39.3496) -> (-27.4474, -39.6671) centre (-23.3723, -41.1407) ccw
  arc A2092 (-27.7902, -40.2761) -> (-27.4474, -39.6671) centre (-29.4401, -38.9465) ccw
  arc A2093 (-28.3031, -40.7173) -> (-27.7902, -40.2761) centre (-29.2446, -39.1041) ccw
  arc A2094 (-28.9914, -40.9814) -> (-28.3031, -40.7173) centre (-29.455, -38.7436) ccw
  arc A2095 (-29.8501, -41.0694) -> (-28.9914, -40.9814) centre (-29.8501, -36.8359) ccw
  arc A2096 (-30.6893, -40.9855) -> (-29.8501, -41.0694) centre (-29.8501, -36.8289) ccw
  arc A2097 (-31.361, -40.7334) -> (-30.6893, -40.9855) centre (-30.2432, -38.7759) ccw
  arc A2098 (-31.8875, -40.2987) -> (-31.361, -40.7334) centre (-30.3681, -38.9946) ccw
  arc A2099 (-32.2946, -39.6735) -> (-31.8875, -40.2987) centre (-29.7393, -38.455) ccw
  arc A2100 (-32.6657, -38.3841) -> (-32.2946, -39.6735) centre (-28.6007, -37.912) ccw
  arc A2101 (-32.5049, -37.2459) -> (-32.6657, -38.3841) centre (-30.4112, -38.1222) ccw
  arc A2102 (-31.8019, -36.3145) -> (-32.5049, -37.2459) centre (-30.331, -38.1558) ccw
  arc A2103 (-30.6003, -35.6255) -> (-31.8019, -36.3145) centre (-28.9717, -39.8574) ccw
  arc A2104 (-30.6003, -35.6255) -> (-29.7645, -35.2907) centre (-42.4988, -4.7076) ccw
  arc A2105 (-29.7645, -35.2907) -> (-29.7383, -35.1709) centre (-29.7932, -35.2216) ccw
  arc A2106 (-29.7383, -35.1709) -> (-29.9156, -35.12) centre (-29.8688, -35.2914) ccw
  arc A2107 (-29.9156, -35.12) -> (-30.8266, -35.3804) centre (-19.4246, -73.5425) ccw
  arc A2108 (-28.0815, -36.1366) -> (-28.5708, -35.7902) centre (-29.4447, -37.5437) ccw
  arc A2109 (-27.6578, -36.6512) -> (-28.0815, -36.1366) centre (-30.1481, -38.2698) ccw
  arc A2110 (-27.2758, -37.3697) -> (-27.6578, -36.6512) centre (-31.5499, -39.1809) ccw
  arc A2111 (-26.9119, -38.3426) -> (-27.2758, -37.3697) centre (-38.4359, -42.0988) ccw
  arc A2112 (-26.9119, -38.3426) -> (-26.8627, -38.4431) centre (-26.5309, -38.2184) ccw
  arc A2113 (-26.8627, -38.4431) -> (-26.8194, -38.4426) centre (-26.8412, -38.4286) ccw
  arc A2114 (-26.8194, -38.4426) -> (-26.7854, -38.3447) centre (-27.0043, -38.3236) ccw
  arc A2115 (-26.7854, -38.3447) -> (-26.7711, -38.124) centre (-30.2739, -38.0079) ccw
  arc A2116 (-26.7711, -38.124) -> (-26.9492, -37.2487) centre (-28.6976, -38.0601) ccw
  arc A2117 (-26.9492, -37.2487) -> (-27.5374, -36.3142) centre (-30.8949, -39.0798) ccw
  arc A2118 (-27.5374, -36.3142) -> (-28.3076, -35.5955) centre (-30.6514, -38.8793) ccw
  arc A2119 (-28.3076, -35.5955) -> (-29.0282, -35.3839) centre (-28.9726, -36.5273) ccw
  arc A2120 (-29.0282, -35.3839) -> (-29.0685, -35.43) centre (-29.0261, -35.4263) ccw
  arc A2121 (-29.0685, -35.43) -> (-29.0284, -35.5098) centre (-28.9482, -35.4195) ccw
  arc A2122 (-29.0284, -35.5098) -> (-28.8509, -35.6387) centre (-28.2864, -34.6746) ccw
  arc A2123 (-28.8509, -35.6387) -> (-28.5708, -35.7902) centre (-26.4613, -31.5574) ccw
  arc A2124 (-30.5938, -36.9036) -> (-30.9535, -37.1438) centre (-29.1294, -39.486) ccw
  arc A2125 (-30.9535, -37.1438) -> (-31.2251, -37.4072) centre (-29.8784, -38.5242) ccw
  arc A2126 (-31.2251, -37.4072) -> (-31.3966, -37.6791) centre (-30.2674, -38.2016) ccw
  arc A2127 (-31.3966, -37.6791) -> (-31.4576, -37.945) centre (-30.7975, -37.9563) ccw
  arc A2128 (-31.4576, -37.945) -> (-31.4112, -37.978) centre (-31.4231, -37.9456) ccw
  arc A2129 (-31.4112, -37.978) -> (-31.2817, -37.9092) centre (-31.6, -37.466) ccw
  arc A2130 (-31.2817, -37.9092) -> (-31.0868, -37.7477) centre (-32.3502, -36.4213) ccw
  arc A2131 (-31.0868, -37.7477) -> (-30.8535, -37.5112) centre (-34.763, -33.888) ccw
  arc A2132 (-30.2444, -37.001) -> (-30.8535, -37.5112) centre (-28.5354, -39.6596) ccw
  arc A2133 (-29.7084, -36.879) -> (-30.2444, -37.001) centre (-29.8082, -37.6796) ccw
  arc A2134 (-29.223, -37.129) -> (-29.7084, -36.879) centre (-29.8064, -37.6656) ccw
  arc A2135 (-28.7706, -37.7707) -> (-29.223, -37.129) centre (-31.4604, -39.1866) ccw
  arc A2136 (-28.6034, -38.4226) -> (-28.7706, -37.7707) centre (-30.0582, -38.4485) ccw
  arc A2137 (-28.7719, -39.0196) -> (-28.6034, -38.4226) centre (-29.6774, -38.4417) ccw
  arc A2138 (-29.2532, -39.4462) -> (-28.7719, -39.0196) centre (-29.7612, -38.3883) ccw
  arc A2139 (-29.9519, -39.6217) -> (-29.2532, -39.4462) centre (-30.032, -37.8242) ccw
  line L98 (-29.9519, -39.6217) -> (-30.8417, -39.6614)
  line L99 (-30.8417, -39.6614) -> (-30.0129, -39.7631)
  arc A2140 (-30.0129, -39.7631) -> (-28.9917, -39.5941) centre (-29.7895, -37.9428) ccw
  arc A2141 (-28.9917, -39.5941) -> (-28.3363, -38.9059) centre (-29.5789, -38.3787) ccw
  arc A2142 (-28.3363, -38.9059) -> (-28.2998, -37.961) centre (-29.5631, -38.3854) ccw
  arc A2143 (-28.2998, -37.961) -> (-28.892, -37.1212) centre (-30.0026, -38.5331) ccw
  arc A2144 (-28.892, -37.1212) -> (-29.3926, -36.773) centre (-32.102, -41.202) ccw
  arc A2145 (-29.3926, -36.773) -> (-29.7573, -36.6448) centre (-29.8744, -37.5606) ccw
  arc A2146 (-29.7573, -36.6448) -> (-30.1183, -36.6846) centre (-29.8553, -37.4111) ccw
  arc A2147 (-30.1183, -36.6846) -> (-30.5938, -36.9036) centre (-29.0598, -39.6087) ccw
  arc A2148 (-31.4614, -38.6524) -> (-31.4418, -38.8193) centre (-30.7416, -38.6524) ccw
  arc A2149 (-31.4418, -38.8193) -> (-31.3837, -38.9862) centre (-30.5882, -38.6159) ccw
  arc A2150 (-31.3837, -38.9862) -> (-31.2982, -39.1283) centre (-30.6728, -38.6552) ccw
  arc A2151 (-31.2982, -39.1283) -> (-31.197, -39.2204) centre (-31.0012, -38.9036) ccw
  arc A2152 (-31.197, -39.2204) -> (-30.952, -39.3299) centre (-30.6665, -38.3621) ccw
  arc A2153 (-30.952, -39.3299) -> (-30.8516, -39.2678) centre (-30.9296, -39.2539) ccw
  arc A2154 (-30.8516, -39.2678) -> (-30.8864, -39.0708) centre (-31.1384, -39.2169) ccw
  arc A2155 (-30.8864, -39.0708) -> (-31.1098, -38.7287) centre (-34.224, -41.0058) ccw
  arc A2156 (-31.1098, -38.7287) -> (-31.3087, -38.4672) centre (-38.1112, -43.8482) ccw
  arc A2157 (-31.3087, -38.4672) -> (-31.3959, -38.4129) centre (-31.4281, -38.5617) ccw
  arc A2158 (-31.3959, -38.4129) -> (-31.4487, -38.4503) centre (-31.4052, -38.4558) ccw
  arc A2159 (-31.4487, -38.4503) -> (-31.4614, -38.6524) centre (-29.8384, -38.6524) ccw
  arc A2160 (-30.6679, 40.8071) -> (-31.3549, 40.2563) centre (-29.8065, 39.0286) ccw
  arc A2161 (-31.3549, 40.2563) -> (-31.5901, 39.5459) centre (-30.5016, 39.5797) ccw
  arc A2162 (-31.5901, 39.5459) -> (-31.3191, 38.7844) centre (-30.2688, 39.587) ccw
  arc A2163 (-31.3191, 38.7844) -> (-30.5836, 38.1003) centre (-28.9483, 40.5961) ccw
  arc A2164 (-30.5836, 38.1003) -> (-29.6091, 37.8817) centre (-29.8054, 39.2881) ccw
  arc A2165 (-29.6091, 37.8817) -> (-28.7184, 38.3552) centre (-29.8124, 39.3383) ccw
  arc A2166 (-28.7184, 38.3552) -> (-28.3085, 39.3192) centre (-29.9207, 39.4357) ccw
  arc A2167 (-28.3085, 39.3192) -> (-28.5728, 40.3377) centre (-29.9467, 39.4376) ccw
  arc A2168 (-28.5728, 40.3377) -> (-28.9831, 40.7911) centre (-30.224, 39.2558) ccw
  arc A2169 (-28.9831, 40.7911) -> (-29.4639, 41.0234) centre (-29.7202, 39.8791) ccw
  arc A2170 (-29.4639, 41.0234) -> (-30.0239, 41.027) centre (-29.7523, 39.736) ccw
  arc A2171 (-30.0239, 41.027) -> (-30.6679, 40.8071) centre (-29.4477, 38.2877) ccw
  arc A2172 (-28.647, 39.6278) -> (-28.8728, 40.1693) centre (-30.2062, 39.2955) ccw
  arc A2173 (-28.6605, 39.0882) -> (-28.647, 39.6278) centre (-29.7808, 39.3862) ccw
  arc A2174 (-28.9152, 38.6229) -> (-28.6605, 39.0882) centre (-29.7354, 39.3741) ccw
  arc A2175 (-29.3724, 38.2906) -> (-28.9152, 38.6229) centre (-29.9597, 39.5795) ccw
  arc A2176 (-29.906, 38.1363) -> (-29.3724, 38.2906) centre (-30.1634, 40.0266) ccw
  arc A2177 (-30.3546, 38.1935) -> (-29.906, 38.1363) centre (-30.0238, 39.0012) ccw
  arc A2178 (-30.7406, 38.4744) -> (-30.3546, 38.1935) centre (-29.9746, 39.1212) ccw
  arc A2179 (-31.0873, 38.9929) -> (-30.7406, 38.4744) centre (-28.6089, 40.2745) ccw
  arc A2180 (-31.2705, 39.3977) -> (-31.0873, 38.9929) centre (-27.2952, 40.9539) ccw
  arc A2181 (-31.3027, 39.6482) -> (-31.2705, 39.3977) centre (-30.7863, 39.5872) ccw
  arc A2182 (-31.2124, 39.8782) -> (-31.3027, 39.6482) centre (-30.8197, 39.5912) ccw
  arc A2183 (-30.9445, 40.2023) -> (-31.2124, 39.8782) centre (-28.3534, 37.7884) ccw
  arc A2184 (-30.4236, 40.5867) -> (-30.9445, 40.2023) centre (-29.6572, 39.003) ccw
  arc A2185 (-29.8407, 40.7155) -> (-30.4236, 40.5867) centre (-29.8613, 39.4248) ccw
  arc A2186 (-29.2945, 40.5659) -> (-29.8407, 40.7155) centre (-29.8589, 39.577) ccw
  arc A2187 (-28.8728, 40.1693) -> (-29.2945, 40.5659) centre (-29.908, 39.4909) ccw
  arc A2188 (-8.2954, 16.823) -> (-8.5283, 16.5527) centre (-6.5947, 15.1222) ccw
  arc A2189 (-8.5283, 16.5527) -> (-8.7252, 16.2443) centre (-6.389, 14.97) ccw
  arc A2190 (-8.7252, 16.2443) -> (-8.8614, 15.9448) centre (-6.7303, 15.1562) ccw
  arc A2191 (-8.8614, 15.9448) -> (-8.9039, 15.7075) centre (-8.22, 15.7075) ccw
  arc A2192 (-8.9039, 15.7075) -> (-8.5627, 14.8613) centre (-7.684, 15.7075) ccw
  arc A2193 (-8.5627, 14.8613) -> (-7.6557, 14.3037) centre (-7.0313, 16.336) ccw
  arc A2194 (-7.6557, 14.3037) -> (-6.5876, 14.2539) centre (-7.0247, 16.3574) ccw
  arc A2195 (-6.5876, 14.2539) -> (-5.8194, 14.7598) centre (-6.8415, 15.4757) ccw
  arc A2196 (-5.8194, 14.7598) -> (-5.5331, 15.3284) centre (-7.6296, 16.0277) ccw
  arc A2197 (-5.5331, 15.3284) -> (-5.4541, 15.9067) centre (-7.0282, 15.8272) ccw
  arc A2198 (-5.4541, 15.9067) -> (-5.5911, 16.4544) centre (-6.9119, 15.833) ccw
  arc A2199 (-5.5911, 16.4544) -> (-5.9293, 16.9356) centre (-7.1385, 15.7264) ccw
  arc A2200 (-5.9293, 16.9356) -> (-6.4717, 17.2989) centre (-7.1189, 15.746) ccw
  arc A2201 (-6.4717, 17.2989) -> (-7.0872, 17.4069) centre (-7.0195, 15.9845) ccw
  arc A2202 (-7.0872, 17.4069) -> (-7.7163, 17.2416) centre (-7.0128, 15.8442) ccw
  arc A2203 (-7.7163, 17.2416) -> (-8.2954, 16.823) centre (-6.7048, 15.2323) ccw
  arc A2204 (-5.9638, 16.0846) -> (-6.3826, 16.7733) centre (-7.3319, 15.7243) ccw
  arc A2205 (-6.0046, 15.2998) -> (-5.9638, 16.0846) centre (-7.2112, 15.7561) ccw
  arc A2206 (-6.4925, 14.688) -> (-6.0046, 15.2998) centre (-7.1983, 15.7512) ccw
  arc A2207 (-7.2586, 14.4568) -> (-6.4925, 14.688) centre (-7.2586, 15.842) ccw
  arc A2208 (-7.9175, 14.7142) -> (-7.2586, 14.4568) centre (-7.2586, 15.4285) ccw
  arc A2209 (-8.3167, 15.3833) -> (-7.9175, 14.7142) centre (-6.9866, 15.7234) ccw
  arc A2210 (-8.2984, 16.1898) -> (-8.3167, 15.3833) centre (-6.868, 15.7537) ccw
  arc A2211 (-7.8572, 16.7976) -> (-8.2984, 16.1898) centre (-7.1961, 15.8538) ccw
  arc A2212 (-7.3915, 17.082) -> (-7.8572, 16.7976) centre (-5.3643, 13.2385) ccw
  arc A2213 (-7.0695, 17.1589) -> (-7.3915, 17.082) centre (-7.0805, 16.4924) ccw
  arc A2214 (-6.7681, 17.0679) -> (-7.0695, 17.1589) centre (-7.079, 16.5825) ccw
  arc A2215 (-6.3826, 16.7733) -> (-6.7681, 17.0679) centre (-8.3476, 14.602) ccw
  arc A2216 (22.0817, 16.9356) -> (21.6198, 16.0978) centre (23.2989, 15.7184) ccw
  arc A2217 (21.6198, 16.0978) -> (21.6998, 15.1764) centre (23.1038, 15.7625) ccw
  arc A2218 (21.6998, 15.1764) -> (22.2982, 14.4734) centre (23.0973, 15.7598) ccw
  arc A2219 (22.2982, 14.4734) -> (23.2167, 14.2168) centre (23.1981, 15.9221) ccw
  arc A2220 (23.2167, 14.2168) -> (24.204, 14.4638) centre (23.1928, 16.4084) ccw
  arc A2221 (24.204, 14.4638) -> (24.8384, 15.1158) centre (23.5358, 15.7488) ccw
  arc A2222 (24.8384, 15.1158) -> (24.932, 15.9775) centre (23.6832, 15.6771) ccw
  arc A2223 (24.932, 15.9775) -> (24.4716, 16.7992) centre (23.2439, 15.5715) ccw
  arc A2224 (24.4716, 16.7992) -> (23.8801, 17.232) centre (22.7796, 15.1072) ccw
  arc A2225 (23.8801, 17.232) -> (23.2459, 17.4058) centre (23.1562, 15.8344) ccw
  arc A2226 (23.2459, 17.4058) -> (22.6282, 17.301) centre (23.1659, 16.0043) ccw
  arc A2227 (22.6282, 17.301) -> (22.0817, 16.9356) centre (23.2743, 15.743) ccw
  arc A2228 (24.4087, 16.2393) -> (24.0648, 16.6877) centre (22.5359, 15.1589) ccw
  arc A2229 (24.5382, 15.7986) -> (24.4087, 16.2393) centre (23.5636, 15.7518) ccw
  arc A2230 (24.4499, 15.3581) -> (24.5382, 15.7986) centre (23.6159, 15.7543) ccw
  arc A2231 (24.1503, 14.9101) -> (24.4499, 15.3581) centre (22.7774, 16.1526) ccw
  arc A2232 (23.7486, 14.6098) -> (24.1503, 14.9101) centre (23.1825, 15.7859) ccw
  arc A2233 (23.2532, 14.4737) -> (23.7486, 14.6098) centre (23.1278, 15.8997) ccw
  arc A2234 (22.7643, 14.5239) -> (23.2532, 14.4737) centre (23.1393, 15.7692) ccw
  arc A2235 (22.3791, 14.7542) -> (22.7643, 14.5239) centre (23.0295, 15.4046) ccw
  arc A2236 (22.1505, 15.1639) -> (22.3791, 14.7542) centre (22.9873, 15.3624) ccw
  arc A2237 (22.0944, 15.7592) -> (22.1505, 15.1639) centre (24.2495, 15.6619) ccw
  arc A2238 (22.205, 16.3615) -> (22.0944, 15.7592) centre (24.3418, 15.6577) ccw
  arc A2239 (22.4712, 16.794) -> (22.205, 16.3615) centre (23.2468, 16.0184) ccw
  arc A2240 (22.8592, 17.0798) -> (22.4712, 16.794) centre (23.6075, 15.6577) ccw
  arc A2241 (23.24, 17.1605) -> (22.8592, 17.0798) centre (23.1924, 16.4465) ccw
  arc A2242 (23.6344, 17.0319) -> (23.24, 17.1605) centre (23.1839, 16.3194) ccw
  arc A2243 (24.0648, 16.6877) -> (23.6344, 17.0319) centre (22.3029, 14.9259) ccw
  arc A2244 (-21.9874, 11.6757) -> (-23.7081, 9.9429) centre (135.1394, -146.073) ccw
  arc A2245 (-23.7081, 9.9429) -> (-25.1354, 8.4629) centre (56.5052, -68.8403) ccw
  arc A2246 (-25.1354, 8.4629) -> (-26.3694, 7.1553) centre (362.9565, -359.0112) ccw
  arc A2247 (-26.3694, 7.1553) -> (-26.3678, 7.0496) centre (-26.3141, 7.1033) ccw
  arc A2248 (-26.3678, 7.0496) -> (-26.262, 7.0479) centre (-26.314, 7.1034) ccw
  arc A2249 (-26.262, 7.0479) -> (-24.9519, 8.2793) centre (-392.1175, 397.5835) ccw
  arc A2250 (-24.9519, 8.2793) -> (-23.469, 9.7038) centre (-102.0967, 90.0756) ccw
  arc A2251 (-23.469, 9.7038) -> (-21.7328, 11.421) centre (-179.172, 168.8606) ccw
  arc A2252 (-21.7328, 11.421) -> (-20.0148, 13.1566) centre (-190.5627, 180.2508) ccw
  arc A2253 (-20.0148, 13.1566) -> (-18.5884, 14.6376) centre (-106.1473, 97.5447) ccw
  arc A2254 (-18.5884, 14.6376) -> (-17.3509, 15.9484) centre (-466.259, 438.5239) ccw
  arc A2255 (-17.3509, 15.9484) -> (-17.3524, 16.0472) centre (-17.4026, 15.997) ccw
  arc A2256 (-17.3524, 16.0472) -> (-17.4513, 16.0488) centre (-17.4027, 15.9969) ccw
  arc A2257 (-17.4513, 16.0488) -> (-18.7646, 14.8138) centre (404.2629, -433.7201) ccw
  arc A2258 (-18.7646, 14.8138) -> (-20.2484, 13.3902) centre (63.9727, -72.9122) ccw
  arc A2259 (-20.2484, 13.3902) -> (-21.9874, 11.6757) centre (146.5104, -157.4894) ccw
  arc A2260 (-18.704, 10.482) -> (-20.0116, 9.1541) centre (79.2065, -87.2412) ccw
  arc A2261 (-20.0116, 9.1541) -> (-21.0713, 8.0371) centre (26.5144, -36.0482) ccw
  arc A2262 (-21.0713, 8.0371) -> (-21.9418, 7.0899) centre (97.0133, -101.3615) ccw
  arc A2263 (-21.9418, 7.0899) -> (-21.9111, 7.0202) centre (-21.9111, 7.0619) ccw
  arc A2264 (-21.9111, 7.0202) -> (-21.5182, 7.1823) centre (-21.9111, 7.5773) ccw
  arc A2265 (-21.5182, 7.1823) -> (-18.3358, 10.3592) centre (-875.7757, 866.0965) ccw
  arc A2266 (-18.3358, 10.3592) -> (-15.1246, 13.5854) centre (-1235.0734, 1224.6816) ccw
  arc A2267 (-15.1246, 13.5854) -> (-15.125, 13.8198) centre (-15.2424, 13.7024) ccw
  arc A2268 (-15.125, 13.8198) -> (-15.2238, 13.8217) centre (-15.1754, 13.7694) ccw
  arc A2269 (-15.2238, 13.8217) -> (-16.2274, 12.8904) centre (169.6551, -186.4212) ccw
  arc A2270 (-16.2274, 12.8904) -> (-17.3702, 11.8004) centre (31.9023, -38.7164) ccw
  arc A2271 (-17.3702, 11.8004) -> (-18.704, 10.482) centre (80.1504, -88.1831) ccw
  arc A2272 (40.0946, 11.069) -> (39.334, 10.2406) centre (70.2997, -17.4278) ccw
  arc A2273 (39.334, 10.2406) -> (39.3393, 10.0529) centre (39.4359, 10.1496) ccw
  arc A2274 (39.3393, 10.0529) -> (39.5257, 10.049) centre (39.4345, 10.1482) ccw
  arc A2275 (39.5257, 10.049) -> (40.3425, 10.8211) centre (11.4692, 40.5476) ccw
  arc A2276 (40.3425, 10.8211) -> (40.6857, 11.1749) centre (34.5671, 16.7673) ccw
  arc A2277 (40.6857, 11.1749) -> (40.9515, 11.496) centre (37.5367, 14.053) ccw
  arc A2278 (40.9515, 11.496) -> (41.1324, 11.7604) centre (37.9707, 13.728) ccw
  arc A2279 (41.1324, 11.7604) -> (41.1209, 11.8606) centre (41.0636, 11.8033) ccw
  arc A2280 (41.1209, 11.8606) -> (41.0213, 11.8714) centre (41.0644, 11.8041) ccw
  arc A2281 (41.0213, 11.8714) -> (40.7601, 11.6874) centre (43.0116, 8.7685) ccw
  arc A2282 (40.7601, 11.6874) -> (40.4433, 11.4173) centre (43.3547, 8.3236) ccw
  arc A2283 (40.4433, 11.4173) -> (40.0946, 11.069) centre (46.1263, 5.3785) ccw
  arc A2284 (-18.3235, -13.6781) -> (-19.3963, -14.7717) centre (47.9344, -79.7481) ccw
  arc A2285 (-19.3963, -14.7717) -> (-20.2583, -15.6914) centre (11.6897, -44.7706) ccw
  arc A2286 (-20.2583, -15.6914) -> (-20.9492, -16.4598) centre (43.0867, -73.3484) ccw
  arc A2287 (-20.9492, -16.4598) -> (-20.9182, -16.5288) centre (-20.9182, -16.4873) ccw
  arc A2288 (-20.9182, -16.5288) -> (-20.7557, -16.4661) centre (-20.9182, -16.2867) ccw
  arc A2289 (-20.7557, -16.4661) -> (-19.9081, -15.6914) centre (-106.0676, 77.7159) ccw
  arc A2290 (-19.9081, -15.6914) -> (-18.9352, -14.7708) centre (-55.5803, 22.9816) ccw
  arc A2291 (-18.9352, -14.7708) -> (-17.8277, -13.6781) centre (-85.3976, 53.7) ccw
  arc A2292 (-17.8277, -13.6781) -> (-16.755, -12.5845) centre (-84.0857, 52.3918) ccw
  arc A2293 (-16.755, -12.5845) -> (-15.893, -11.6648) centre (-47.8409, 17.4144) ccw
  arc A2294 (-15.893, -11.6648) -> (-15.202, -10.8965) centre (-79.2379, 45.9922) ccw
  arc A2295 (-15.202, -10.8965) -> (-15.233, -10.8274) centre (-15.233, -10.8689) ccw
  arc A2296 (-15.233, -10.8274) -> (-15.3956, -10.8901) centre (-15.233, -11.0696) ccw
  arc A2297 (-15.3956, -10.8901) -> (-16.2431, -11.6648) centre (69.9164, -105.0722) ccw
  arc A2298 (-16.2431, -11.6648) -> (-17.216, -12.5855) centre (19.4291, -50.3378) ccw
  arc A2299 (-17.216, -12.5855) -> (-18.3235, -13.6781) centre (49.2464, -81.0562) ccw
  arc A2300 (-16.0961, -13.6818) -> (-16.4001, -14.0136) centre (-10.3485, -19.2526) ccw
  arc A2301 (-16.4001, -14.0136) -> (-16.614, -14.2919) centre (-14.1223, -15.9855) ccw